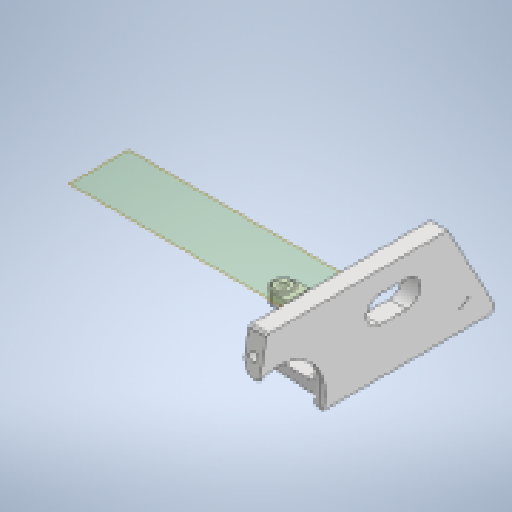
# Autodesk Inventor part: sciana_prawa_nowa
Saved by Autodesk Inventor 2023 (Build 270158000, 158)
## iProperties
Created: 2023-07-07
Part Number: sciana_prawa_nowa
Material: Ogólny
Document SubType Name: Modeling
Designer: Kamil
Density: 1 g/cm^3
Appearance: Domyślna
Author: Kamil
Autodesk Inventor part; units mm, degrees
ref_plane "YZ Plane" through (0, 0, 0) normal (1, 0, 0) x (0, 1, 0)
ref_plane "XZ Plane" through (0, 0, 0) normal (0, 1, 0) x (-1, 0, 0)
ref_plane "XY Plane" through (0, 0, 0) normal (0, 0, 1) x (1, 0, 0)
sketch "Szkic1" plane through (0, 0, 0) normal (1, 0, 0) x (0, 1, 0)
  line L0 (-17.6056, -88.6767) -> (14.5, -71.5061)
  line L1 (14.5, -71.5061) -> (14.5, -4.8975)
  arc A0 (14.5, -4.8975) -> (13.7161, -3.9211) centre (13.5, -4.8975) ccw
  line L2 (13.7161, -3.9211) -> (0.9006, -1.0853)
  arc A1 (0.9006, -1.0853) -> (-0.2326, -2.4602) centre (0.6845, -2.0617) ccw
  arc A2 (-7.376, -23.624) -> (-0.2326, -2.4602) centre (-15.5, -9.0945) ccw
  arc A3 (-20.5, -24.8945) -> (-7.376, -23.624) centre (-15.5, -8.124) ccw
  line L3 (-20.5, -24.8945) -> (-20.5, -86.8879)
  arc A4 (-20.5, -86.8879) -> (-17.6056, -88.6767) centre (-18.5, -86.8879) ccw
  line L4 (-16.7851, -50.8138) -> (-12.7851, -50.8138)
  line L5 (-12.7851, -50.8138) -> (-12.7851, -57.2138)
  line L6 (-12.7851, -57.2138) -> (-16.7851, -57.2138)
  line L7 (-16.7851, -57.2138) -> (-16.7851, -50.8138)
  point P0 (0, 0)
  point P1 (-20.5, -2.4444)
  constraints: 16 end point, 10 point on circle, 5 centre point
extrude "Wyciągnięcie proste1" add sketch "Szkic1" against normal blind 6.5
sketch "Szkic2" plane through (0, -20.5, -86.8879) normal (0, -1, 0) x (1, 0, 0)
  line L0 (0, 0) -> (-6.5, 0)
  line L1 (0, 61.9933) -> (0, 0)
  line L2 (-6.5, 61.9933) -> (0, 61.9933)
  line L3 (-6.5, 58.2191) -> (-6.5, 61.9933)
  line L4 (-6.5, 58.2191) -> (-25.1514, 57.1202)
  arc A0 (-25.1514, 57.1202) -> (-28.4014, 49.274) centre (-25.1514, 52.524) ccw
  line L5 (-28.4014, 49.274) -> (-8.5846, 29.4572)
  arc A1 (-8.5846, 29.4572) -> (-6.5, 28.1275) centre (-4.9489, 32.8582) ccw
  line L6 (-6.5, 0) -> (-6.5, 28.1275)
  line L7 (-3.5, 32.4699) -> (-3.5, 31.874)
  arc A2 (-3.4489, 32.874) -> (-3.5, 32.4699) centre (-4.9489, 32.8582) ccw
  line L8 (-3.4489, 31.874) -> (-3.4489, 32.874)
  line L9 (-3.5, 31.874) -> (-3.4489, 31.874)
  circle A3 centre (-25.1514, 52.524) radius 1.5
  line L10 (-6.5, 28.1275) -> (-6.5, 58.2191)
  line L11 (-6.5, 0) -> (-6.5, 61.9933) projected
  point P0 (0, 86.8879)
  point P1 (0, 61.9933)
  constraints: 22 end point, 6 point on circle, 4 centre point, 1 collinear
extrude "Wyciągnięcie proste2" add sketch "Szkic2" against normal blind 3.7 contours A1 L5 A0 L4 L10
sketch "Szkic3" plane through (0, -16.8, -86.8879) normal (0, 1, 0) x (1, 0, 0)
  circle A0 centre (-25.1514, -52.524) radius 1.5 projected
  circle A1 centre (-25.1514, -52.524) radius 4.5962
  point P0 (0, -86.8879)
  constraints: 1 centre point, 1 coincident
extrude "Wyciągnięcie proste3" add sketch "Szkic3" along normal blind 1.5
sketch "Szkic4" plane through (-25.1514, -15.3, -34.3638) normal (0, 1, 0) x (1, 0, 0)
  circle A0 centre (0, 0) radius 3
  circle A1 centre (0, 0) radius 1.5 projected
  line L0 (-1.7321, -3) -> (-3.4641, 0)
  line L1 (-3.4641, 0) -> (-1.7321, 3)
  line L2 (-1.7321, 3) -> (1.7321, 3)
  line L3 (1.7321, 3) -> (3.4641, 0)
  line L4 (3.4641, 0) -> (1.7321, -3)
  line L5 (1.7321, -3) -> (-1.7321, -3)
  point P0 (25.1514, -34.3638)
  point P1 (0, -3)
  dimension "d6" = 6
  constraints: 12 end point, 1 coincident, 1 midpoint, 1 vertical alignment, 15 other
extrude "Wyciągnięcie proste4" cut sketch "Szkic4" against normal blind 3 contours A0 | A0 L3 L4 | A0 L2 L3 | L4 L5 A0 | A0 L1 L2 | L5 L0 A0 | A0 L0 L1 | A1
sketch "Szkic5" plane through (0, -20.5, -86.8879) normal (0, -1, 0) x (1, 0, 0)
  line L0 (0, 61.9933) -> (0, 0) projected
  line L1 (0, 0) -> (-6.5, 0) projected
  line L2 (0, 34) -> (-5, 34) construction
  line L3 (0, 29.674) -> (-6.5, 29.674) construction
  line L4 (0, 36.074) -> (-6.5, 36.074) construction
  line L5 (-3.25, 29.674) -> (-3.25, 36.074) construction
  circle A0 centre (-5, 32.874) radius 1.5
  point P0 (0, 86.8879)
  dimension "d9" = 5
  dimension "d10" = 3
  constraints: 4 end point, 2 midpoint, 1 centre point, 1 perpendicular, 1 point on line
  measures "d9" distance of L2.start L2.end
  measures "d10" diameter of A0
extrude "Wyciągnięcie proste5" cut sketch "Szkic5" against normal blind 15
sketch "Szkic6" plane through (0, -16.7851, -50.8138) normal (0, 1, 0) x (1, 0, 0)
  circle A0 centre (-5, 3.2) radius 1.5 projected
  circle A1 centre (-5, 3.2) radius 3
  line L0 (-3.2679, 6.2) -> (-1.5359, 3.2)
  line L1 (-1.5359, 3.2) -> (-3.2679, 0.2)
  line L2 (-3.2679, 0.2) -> (-6.7321, 0.2)
  line L3 (-6.7321, 0.2) -> (-8.4641, 3.2)
  line L4 (-8.4641, 3.2) -> (-6.7321, 6.2)
  line L5 (-6.7321, 6.2) -> (-3.2679, 6.2)
  line L6 (-6.5, 3.2) -> (-6.5, 6.4) projected
  line L7 (-6.5, 0) -> (-6.5, 3.2) projected
  line L8 (0, 6.4) -> (0, 0) projected
  line L9 (0, 6.4) -> (-6.5, 6.4) projected
  line L10 (-6.5, 3.2) -> (-6.5, 6.4) projected
  circle A2 centre (-5, 3.2) radius 1.5 projected
  line L11 (-6.5, 0) -> (-6.5, 3.2) projected
  line L12 (0, 0) -> (-6.5, 0) projected
  point P0 (0, -50.8138)
  point P1 (-5, 6.2)
  point P2 (-6.5, 6.2)
  point P3 (-6.5, 0.2)
  dimension "d13" = 6
  constraints: 12 end point, 2 coincident, 2 horizontal alignment, 1 midpoint, 1 vertical alignment, 15 other
extrude "Wyciągnięcie proste6" add sketch "Szkic6" along normal up to surface (4 mm away) contours L5 L6 L9 L8 L12 L7 L2 L1 L0
sketch "Szkic7" plane through (0, 0, 0) normal (1, 0, 0) x (0, 0, -1)
  arc A0 (23.624, -7.376) -> (2.4602, -0.2326) centre (9.0945, -15.5) ccw projected
  arc A1 (24.8945, -20.5) -> (23.624, -7.376) centre (8.124, -15.5) ccw projected
  circle A2 centre (8.124, -15.5) radius 17.75
  point P0 (0, 0)
  dimension "d16" = 35.5
  constraints: 1 centre point, 1 coincident
  measures "d16" diameter of A2
extrude "Wyciągnięcie proste7" cut sketch "Szkic7" against normal through all
fillet "Zaokrąglenie1" radius 5 2 edges at (-6.5, -18.0257, -25.6934) (-6.5, -0.6621, -17.8657)
sketch "Szkic8" plane through (-5, -16.7851, -54.0138) normal (0, 1, 0) x (1, 0, 0)
  line L0 (-1.5, -3) -> (1.7321, -3) projected
  line L1 (1.7321, -3) -> (3.4641, 0) projected
  line L2 (3.4641, 0) -> (1.7321, 3) projected
  line L3 (1.7321, 3) -> (-1.5, 3) projected
  line L4 (-1.5, 0) -> (-1.5, 3) projected
  circle A0 centre (0, 0) radius 1.5 projected
  line L5 (-1.5, -3) -> (-1.5, 0) projected
  point P0 (5, -54.0138)
  constraints: 1 horizontal alignment
extrude "Wyciągnięcie proste8" cut sketch "Szkic8" against normal up to surface (0.0149 mm away)
fillet "Zaokrąglenie2" radius 3.5 2 edges at (-6.3716, -16.8, -29.709) (-6.5, -16.8, -40.9254)
fillet "Zaokrąglenie3" radius 2 1 edges at (-6.5, -16.8, -57.8871)
sketch "Szkic9" plane through (-6.5, 13.7161, -3.9211) normal (0, 0.2160502, 0.9763823) x (1, 0, 0)
  line L0 (6.5, 0) -> (0, 0) projected
  line L1 (3.25, 0) -> (3.25, -7.22)
  circle A0 centre (3.25, -7.22) radius 1.5
  point P0 (6.5, -14.2393)
  dimension "d24" = 7.22
  dimension "d25" = 3
  constraints: 2 end point, 1 centre point, 1 coincident, 1 midpoint, 1 perpendicular
  measures "d24" distance of L1.start L1.end
  measures "d25" diameter of A0
extrude "Wyciągnięcie proste9" cut sketch "Szkic9" against normal blind 15
sketch "Szkic10" plane through (0, -17.6056, -88.6767) normal (0, 0.4716076, -0.8818085) x (-1, 0, 0)
  line L0 (0, 36.4088) -> (6.5, 36.4088) projected
  line L1 (3.2503, 36.4088) -> (3.2503, 10.0668) construction
  line L2 (6.5, 11.5565) -> (6.5, 16.5828) construction
  circle A0 centre (3.2503, 10.0668) radius 1.5
  point P0 (0, 57.3454)
  point P1 (3.25, 36.4088)
  dimension "d28" = 26.342
  dimension "d29" = 3
  constraints: 2 end point, 1 centre point, 1 coincident, 1 midpoint, 1 parallel, 1 point on line
  measures "d28" distance of L1.start L1.end
  measures "d29" diameter of A0
extrude "Wyciągnięcie proste10" cut sketch "Szkic10" against normal blind 15
ref_plane "Płaszczyzna konstrukcyjna1" through (0, -19.9636, -84.2677) normal (0, 0.4716076, -0.8818085) x (-1, 0, 0)
sketch "Szkic11" plane through (0, -19.9636, -84.2677) normal (0, 0.4716076, -0.8818085) x (-1, 0, 0)
  circle A0 centre (3.2503, 10.0668) radius 1.5 projected
  circle A1 centre (3.2503, 10.0668) radius 2.85
  circle A2 centre (3.2503, 10.0668) radius 1.5 projected
  line L0 (1.6049, 7.2168) -> (-0.0406, 10.0668)
  line L1 (-0.0406, 10.0668) -> (1.6049, 12.9168)
  line L2 (1.6049, 12.9168) -> (4.8957, 12.9168)
  line L3 (4.8957, 12.9168) -> (6.5412, 10.0668)
  line L4 (6.5412, 10.0668) -> (4.8957, 7.2168)
  line L5 (4.8957, 7.2168) -> (1.6049, 7.2168)
  line L6 (3.2503, 7.2168) -> (9, 7)
  line L7 (3.2503, 12.9168) -> (9.7576, 12.9168)
  line L8 (9.7576, 12.9168) -> (9, 7)
  point P0 (0, 57.3454)
  dimension "d33" = 5.7
  constraints: 18 end point, 2 coincident, 2 midpoint, 1 horizontal, 1 point on line, 1 vertical alignment, 15 other
extrude "Wyciągnięcie proste11" cut sketch "Szkic11" against normal blind 4 contours A0 | A1 | A1 L3 L4 | A1 L2 L3 | L3 L7 L8 L6 L5 L4 | L4 L5 A1 | A1 L1 L2 | L5 L0 A1 | A1 L0 L1
sketch "Szkic12" plane through (0, 0, 0) normal (1, 0, 0) x (0, 0, -1)
  line L0 (48.1377, 2.65) -> (54.2377, 2.65) projected
  line L1 (42.2468, -1.3) -> (60.0268, -1.3) projected
  line L2 (46.1877, 6.675) -> (56.1877, 6.675)
  line L3 (56.1877, 6.675) -> (56.1877, -3.325)
  line L4 (56.1877, -3.325) -> (46.1877, -3.325)
  line L5 (46.1877, -3.325) -> (46.1877, 6.675)
  line L6 (46.1877, 6.675) -> (56.1877, -3.325) construction
  line L7 (56.1877, 6.675) -> (46.1877, -3.325) construction
  point P0 (0, 0)
  point P1 (51.1877, 1.675)
  dimension "d37" = 10
  dimension "d38" = 10
  constraints: 12 end point, 2 midpoint, 2 parallel, 1 horizontal, 1 perpendicular
  measures "d37" distance of L3.end L4.end
  measures "d38" distance of L2.end L3.end
extrude "Wyciągnięcie proste12" cut sketch "Szkic12" against normal blind 7
sketch "Szkic13" plane through (0, 0, 0) normal (1, 0, 0) x (0, 0, -1)
  line L0 (46.1877, -3.325) -> (46.1877, 6.675) projected
  line L1 (56.1877, 6.675) -> (56.1877, -3.325) projected
  circle A0 centre (46.1877, 1.675) radius 5
  circle A1 centre (56.1877, 1.675) radius 5
  point P0 (0, 0)
  constraints: 2 midpoint, 6 other
extrude "Wyciągnięcie proste13" cut sketch "Szkic13" against normal blind 7 contours A0 L0 | A1 L1 picked at (44.5332, 1.4741) picked at (57.95, 3.1431)
ref_plane "Płaszczyzna konstrukcyjna2" through (-49.4, 9, -62.7671) normal (0, -1, 0) x (1, 0, 0)
sketch "Szkic14" plane through (-49.4, 9, -62.7671) normal (0, -1, 0) x (1, 0, 0)
  circle A0 centre (31.9, 35.0075) radius 1.5 projected
  circle A1 centre (31.9, 35.0075) radius 4
  line L0 (42.9, 57.8696) -> (42.9, -8.7389) projected
  line L1 (31.9, 39.0075) -> (42.9, 39.0075)
  line L2 (42.9, 60.4432) -> (42.9, 31.9997) projected
  line L3 (31.9, 31.0075) -> (42.9, 31.0075)
  line L4 (42.9, 31.9997) -> (42.9, 11.7533) projected
  point P0 (49.4, 62.7671)
  dimension "d43" = 8
  constraints: 4 end point, 2 point on circle, 2 point on line, 1 centre point, 1 coincident, 1 parallel, 1 perpendicular
  measures "d43" diameter of A1
extrude "Wyciągnięcie proste14" add sketch "Szkic14" along normal blind 5
sketch "Szkic15" plane through (-49.4, 9, -62.7671) normal (0, 1, 0) x (1, 0, 0)
  line L0 (31.9, -31.0075) -> (42.9, -31.0075) projected
  arc A0 (31.9, -31.0075) -> (31.9, -39.0075) centre (31.9, -35.0075) ccw projected
  line L1 (42.9, -39.0075) -> (31.9, -39.0075) projected
  line L2 (42.9, -31.0075) -> (42.9, -39.0075) projected
  circle A1 centre (31.9, -35.0075) radius 1.5 projected
  circle A2 centre (31.9, -35.0075) radius 3.5
  point P0 (49.4, -62.7671)
  dimension "d46" = 7
  constraints: 1 centre point, 1 coincident
  measures "d46" diameter of A2
extrude "Wyciągnięcie proste15" cut sketch "Szkic15" against normal blind 0.5 contours L0 L2 L1 A0
chamfer "Faza1" distance 0.5 angle 45 1 edges at (-21, 9, -27.7596)
